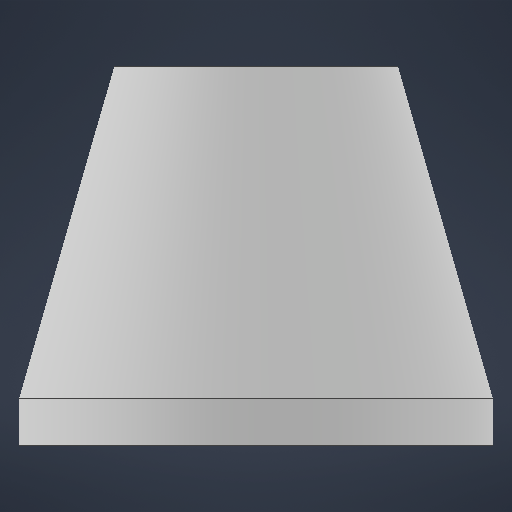
# Autodesk Inventor part: spacer
Saved by Autodesk Inventor 2026 (Build 300175000, 175)
## iProperties
Created: 2026-02-13
Part Number: spacer
Material: 一般
Document SubType Name: Modeling
Designer: numai
Density: 1 g/cm^3
Appearance: 既定
Author: numai
Autodesk Inventor part; units mm, degrees
ref_plane "YZ Plane" through (0, 0, 0) normal (1, 0, 0) x (0, 1, 0)
ref_plane "XZ Plane" through (0, 0, 0) normal (0, 1, 0) x (-1, 0, 0)
ref_plane "XY Plane" through (0, 0, 0) normal (0, 0, 1) x (1, 0, 0)
sketch "スケッチ1" plane through (0, 0, 0) normal (1, 0, 0) x (0, 1, 0)
  line L0 (1.25, 8) -> (1.25, 0)
  line L1 (1.25, 0) -> (5, 0)
  line L2 (5, 0) -> (5, 1)
  line L3 (5, 1) -> (3, 8)
  line L4 (3, 8) -> (1.25, 8)
  line L5 (0, -1.6) -> (0, 9.6) projected
  line L6 (4, 0) -> (1.25, 0.2)
  point P0 (0, 0)
  dimension "d0" = 8
  dimension "d1" = 1
  dimension "d3" = 1.25
  dimension "d4" = 5
  dimension "d6" = 3
  dimension "d7" = 1
  dimension "d8" = 0.2
  constraints: 12 end point, 2 perpendicular, 2 point on line, 1 horizontal, 1 horizontal alignment, 1 vertical
  measures "d0" distance of L0.start L0.end
  measures "d1" distance of L1.end L2.end
  measures "d3" distance from line of point (0, 0) L0
  measures "d4" distance from line of point (0, 0) L2
  measures "d6" horizontal distance of point (0, 0) L3.end
  measures "d7" distance from line of L2 L6.start
  measures "d8" distance of L0.end L6.end
revolve "回転1" add sketch "スケッチ1" angle 360 about axis through (0, 0, -10) along (0, 0, 1)
